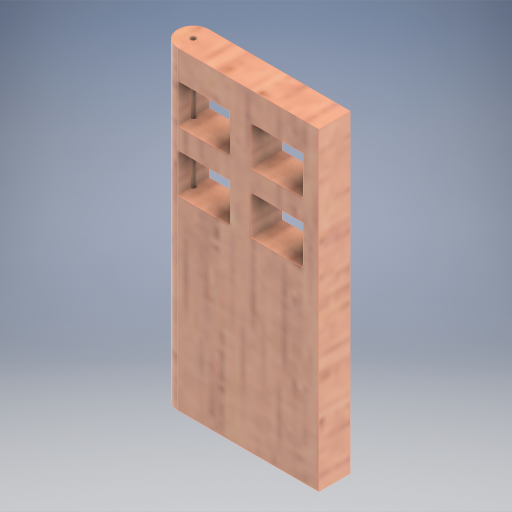
# Autodesk Inventor part: dvere
Saved by Autodesk Inventor 2023 (Build 270158000, 158)
## iProperties
Created: 2022-10-19
Part Number: dvere
Material: Dřevo (dub)
Document SubType Name: Modeling
Designer: zak
Density: 0.76 g/cm^3
Appearance: Dub zimní – přírodní – střední lesk
Mass: 4.42799 g
Surface Area: 42.6781 cm^2
Volume: 5.82631 cm^3
Author: zak
Autodesk Inventor part; units mm, degrees
ref_plane "YZ Plane" through (0, 0, 0) normal (1, 0, 0) x (0, 1, 0)
ref_plane "XZ Plane" through (0, 0, 0) normal (0, 1, 0) x (-1, 0, 0)
ref_plane "XY Plane" through (0, 0, 0) normal (0, 0, 1) x (1, 0, 0)
sketch "Náčrt1" plane through (0, 0, 0) normal (0, 0, 1) x (1, 0, 0)
  line L0 (-15, -30) -> (15, -30)
  line L1 (15, -30) -> (15, 30)
  line L2 (15, 30) -> (-15, 30)
  line L3 (-15, 30) -> (-15, -30)
  line L4 (-15, -30) -> (15, 30) construction
  line L5 (15, -30) -> (-15, 30) construction
  line L6 (0, 30) -> (0, 0)
  line L7 (-15, 15) -> (15, 15)
  line L8 (2, 17) -> (12, 17)
  line L9 (12, 17) -> (12, 24.5)
  line L10 (12, 24.5) -> (2, 24.5)
  line L11 (2, 24.5) -> (2, 17)
  line L12 (-2, 17) -> (-12, 17)
  line L13 (-12, 17) -> (-12, 24.5)
  line L14 (-12, 24.5) -> (-2, 24.5)
  line L15 (-2, 24.5) -> (-2, 17)
  line L16 (2, 13) -> (12, 13)
  line L17 (12, 13) -> (12, 5.5)
  line L18 (12, 5.5) -> (2, 5.5)
  line L19 (2, 5.5) -> (2, 13)
  line L20 (-12, 5.5) -> (-2, 5.5)
  line L21 (-12, 13) -> (-12, 5.5)
  line L22 (-2, 13) -> (-12, 13)
  line L23 (-2, 5.5) -> (-2, 13)
  dimension "d0" = 30
  dimension "d1" = 60
  dimension "d2" = 15
  dimension "d3" = 10
  dimension "d4" = 7.5
  dimension "d5" = 2
  dimension "d6" = 2
  constraints: 48 end point, 12 symmetric about line, 4 parallel, 3 midpoint, 3 perpendicular, 2 horizontal, 2 point on line, 1 vertical
  measures "d0" distance of L2.end L1.end
  measures "d1" distance of L1.end L0.end
  measures "d2" distance between parallel lines of L2 L7
  measures "d3" distance of L10.end L9.end
  measures "d4" distance of L9.end L8.end
  measures "d5" distance between parallel lines of L6 L11
  measures "d6" distance between parallel lines of L7 L8
extrude "Vysunutí1" add sketch "Náčrt1" along normal blind 6
sketch "Náčrt2" plane through (15, -30, 0) normal (0, -1, 0) x (1, 0, 0)
  circle A0 centre (-27, 3) radius 2.4
  line L0 (-30, 0) -> (-30, 6) projected
  line L1 (-30, 6) -> (0, 6) projected
  line L2 (-30, 0) -> (0, 0) projected
  line L3 (-27, 0) -> (-27, 6) projected
  point P0 (-15, 0)
  point P1 (-30, 2)
  point P2 (-30, 4)
  dimension "d13" = 4.8
  dimension "d14" = 3
  dimension "d15" = 3
  dimension "d16" = 3
  constraints: 1 centre point, 1 midpoint
  measures "d13" diameter of A0
  measures "d14" distance from line of L0 A0.centre
  measures "d15" distance from line of L1 A0.centre
  measures "d16" distance from line of L2 point (-27, 3)
extrude "Vysunutí2" cut sketch "Náčrt2" against normal blind 4 contours A0 L3 | L3 A0
full round fillet "Plné kulaté zaoblení1" first side at (0.6667, -18.1667, 6) centre faces at (-15, 10, 2) second side at (0.6667, -18.1667, 0)
sketch "Náčrt3" plane through (15, 30, 6) normal (0, 1, 0) x (1, 0, 0)
  arc A0 (-27, 6) -> (-27, 0) centre (-27, 3) ccw projected
  point P0 (-15, 6)
  constraints: 1 coincident
hole "Díra1" at (-12, 30, 3) direction (0, -1, 0) diameter 1 end through all
